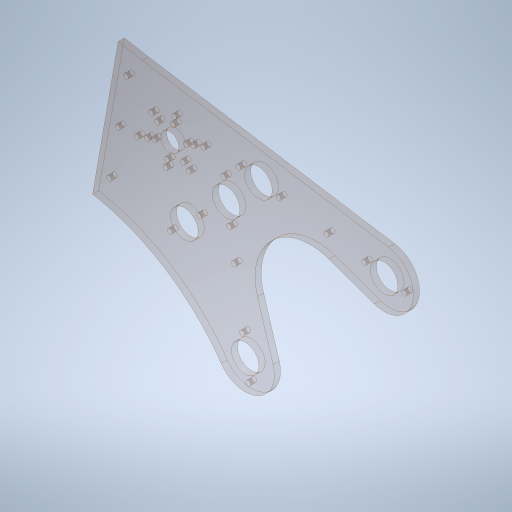
# Autodesk Inventor part: GP7-001
Saved by Autodesk Inventor 2023.4 (Build 274418000, 418)
## iProperties
Created: 2025-02-24
Part Number: GP7-001
Material: Polycarbonate, Smoke
Document SubType Name: Modeling
Designer: dlangdon
Density: 1.2 g/cm^3
Appearance: Polycarbonate - Smoked
Author: dlangdon
Autodesk Inventor part; units mm, degrees
ref_plane "YZ Plane" through (0, 0, 0) normal (1, 0, 0) x (0, 1, 0)
ref_plane "XZ Plane" through (0, 0, 0) normal (0, 1, 0) x (-1, 0, 0)
ref_plane "XY Plane" through (0, 0, 0) normal (0, 0, 1) x (1, 0, 0)
sketch "Sketch1" plane through (0, 0, 0) normal (0, 0, 1) x (1, 0, 0)
  circle A0 centre (71.842, 71.842) radius 50.8 construction
  circle A1 centre (-71.842, -71.842) radius 50.8 construction
  circle A2 centre (0, 0) radius 50.8 construction
  line L0 (-35.921, -35.921) -> (35.921, 35.921) construction
  line L1 (71.842, 71.842) -> (-71.842, -71.842) construction
  line L2 (-4.3707, 6.2419) -> (-4.3707, 50.6116) construction
  line L3 (-226.8798, -122.642) -> (638.5123, -122.642) construction
  circle A3 centre (147.8406, -65.492) radius 57.15 construction
  circle A4 centre (71.842, 71.842) radius 14.2875
  circle A5 centre (-71.842, -71.842) radius 14.2875
  circle A6 centre (-4.3707, 6.2419) radius 57.15 construction
  circle A7 centre (-71.842, -71.842) radius 30.1625 construction
  circle A8 centre (71.842, 71.842) radius 30.1625 construction
  circle A9 centre (-58.1587, 92.2793) radius 14.2875
  line L4 (-58.1587, 92.2793) -> (71.842, 71.842) construction
  circle A10 centre (71.842, 71.842) radius 14.3256 construction
  circle A11 centre (-71.842, -71.842) radius 14.3256 construction
  circle A12 centre (-91.5532, 58.2708) radius 14.2875
  line L5 (-71.842, -71.842) -> (-91.5532, 58.2708) construction
  circle A13 centre (-91.5532, 58.2708) radius 23.8316 construction
  circle A14 centre (-58.1587, 92.2793) radius 23.8316 construction
  line L6 (14.744, 60.1006) -> (61.7538, 43.4167)
  line L7 (-42.9911, -63.0445) -> (-59.0357, -10.4271)
  arc A15 (14.744, 60.1006) -> (-59.0357, -10.4271) centre (-4.3707, 6.2419) ccw
  line L8 (-203.1376, 146.1202) -> (-178.1235, 141.7096)
  line L9 (-178.1235, 141.7096) -> (-204.5875, -8.3751) construction
  line L10 (-204.5875, -8.3751) -> (-229.6016, -3.9645) construction
  line L11 (-229.6016, -3.9645) -> (-203.1376, 146.1202) construction
  line L12 (-245.2736, -92.8451) -> (35.0702, -142.2772) construction
  line L13 (-198.7269, 171.1343) -> (174.1389, 105.388) construction
  line L14 (-198.7269, 171.1343) -> (-245.2736, -92.8451) construction
  circle A16 centre (-149.8604, 82.5886) radius 31.75 construction
  line L15 (-87.9836, 34.7081) -> (-79.4511, -21.6151) construction
  circle A17 centre (12.249, 81.2106) radius 9.525 construction
  line L16 (-190.6305, 143.9149) -> (-217.0945, -6.1698) construction
  line L17 (-195.0412, 118.9008) -> (-212.6839, 18.8443) construction
  circle A18 centre (-149.8604, 82.5886) radius 17.4625 construction
  circle A19 centre (-149.8604, 82.5886) radius 9.525
  circle A20 centre (-58.1587, 92.2793) radius 30.1816 construction
  line L18 (-203.1376, 146.1202) -> (-229.6016, -3.9645)
  arc A21 (61.7538, 43.4167) -> (76.5306, 101.6379) centre (71.842, 71.842) ccw
  arc A22 (-96.6164, -89.047) -> (-42.9911, -63.0445) centre (-71.842, -71.842) ccw
  line L19 (-149.8604, 82.5886) -> (-133.451, 88.5611) construction
  line L20 (-115.5498, 95.0766) -> (-184.1709, 70.1006) construction
  circle A23 centre (-184.1709, 70.1006) radius 4.7625 construction
  line L21 (0, 0) -> (-4.3707, 6.2419) construction
  circle A24 centre (71.842, 71.842) radius 28.6512 construction
  line L22 (64.3298, 44.1932) -> (-61.9049, 78.4917) construction
  line L23 (73.1757, 100.4622) -> (-57.4936, 106.5513) construction
  line L24 (-178.1235, 141.7096) -> (76.5306, 101.6379)
  line L25 (-149.8604, 82.5886) -> (-134.7687, 17.0965) construction
  circle A25 centre (-134.7687, 17.0965) radius 31.75 construction
  circle A26 centre (-134.7687, 17.0965) radius 14.2875
  line L26 (-91.5532, 58.2708) -> (-134.7687, 17.0965) construction
  circle A27 centre (-149.8604, 82.5886) radius 25.4 construction
  arc A28 (-96.6164, -89.047) -> (-229.6016, -3.9645) centre (-265.2541, -206.1602) ccw
  point P0 (-83.7173, 6.5465)
  point P1 (-203.8625, 68.8725)
  point P2 (-203.8625, 68.8725)
  point P3 (-146.828, 99.7858)
  point P4 (-163.2374, 93.8133)
  point P5 (-166.2697, 76.6161)
  point P6 (-152.8927, 65.3914)
  point P7 (-136.4833, 71.3639)
  point P8 (-125.9922, 91.2759)
  point P9 (-145.4497, 107.6027)
  point P10 (-169.3179, 98.9154)
  point P11 (-173.7285, 73.9013)
  point P12 (-154.271, 57.5745)
  point P13 (-130.4028, 66.2618)
  dimension "d7" = 101.6
  dimension "d18" = 47.6631
  dimension "d34" = 34.925
  dimension "d65" = 50.8
  dimension "d3" = 45
  dimension "d4" = 0
  dimension "d8" = 101.6
  dimension "d9" = 28.575
  dimension "d10" = 101.6
  dimension "d11" = 114.3
  dimension "d12" = 114.3
  dimension "d13" = 15.875
  dimension "d14" = 15.875
  dimension "d15" = 131.5974
  dimension "d16" = 28.6512
  dimension "d17" = 131.5974
  dimension "d19" = 47.6631
  dimension "d22" = 25.4
  dimension "d23" = 152.4
  dimension "d26" = 268.0517
  dimension "d27" = 63.5
  dimension "d30" = 200.025
  dimension "d31" = 10
  dimension "d32" = 19.05
  dimension "d33" = 101.6
  dimension "d35" = 19.05
  dimension "d36" = 6.35
  dimension "d40" = 360
  dimension "d44" = 9.525
  dimension "d55" = 80
  dimension "d56" = 7.62
  dimension "d57" = 25.4
  dimension "d58" = 57.3024
  dimension "d59" = 63.5
  dimension "d60" = 67.2084
  dimension "d61" = 59.69
  dimension "d62" = 55
  dimension "d68" = 360
  dimension "d70" = 38.1
  dimension "d71" = 60
  constraints: 54 end point, 25 centre point, 23 coincident, 21 point on circle, 16 tangent, 7 midpoint, 6 equal radius, 5 point on line, 4 collinear, 4 parallel, 2 horizontal, 1 concentric, 1 perpendicular, 1 vertical, 29 other
  measures "d3" angle of L2 L0
  measures "d4" distance between parallel lines of L0 L1
  measures "d8" diameter of A2
  measures "d9" diameter of A4
  measures "d10" diameter of A0
  measures "d11" diameter of A3
  measures "d12" diameter of A6
  measures "d13" radial gap between concentric circles of A5 A7
  measures "d14" radial gap between concentric circles of A4 A8
  measures "d15" distance of L4.start L4.end
  measures "d16" diameter of A10
  measures "d17" distance of L5.start L5.end
  measures "d19" diameter of A14
  measures "d22" distance of L9.end L10.end
  measures "d23" distance of L10.end L8.start
  measures "d26" distance of L13.start L12.start
  measures "d27" diameter of A16
  measures "d30" distance from line of point (0, 0) L9
  measures "d31" angle of L3 L12
  measures "d32" diameter of A17
  measures "d33" distance of L17.start L17.end
  measures "d35" diameter of A19
  measures "d36" radial gap between concentric circles of A14 A20
  measures "d44" diameter of A23
  measures "d55" angle of L1 L21
  measures "d56" distance of L21.start L21.end
  measures "d57" distance between parallel lines of L13 L8
  measures "d58" diameter of A24
  measures "d59" diameter of A25
  measures "d60" distance of L19.start L25.end
  measures "d61" distance of L26.start L26.end
  measures "d62" angle of L15 L26
  measures "d70" distance from line of L9 L19.start
  measures "d71" angle of L9 L20
extrude "Extrusion1" add sketch "Sketch1" along normal blind 6.35
hole "Hole1" at (12.249, 81.2106, 0) at (-195.0412, 118.9008, 0) at (-203.8625, 68.8725, 0) at (-212.6839, 18.8443, 0) at (-133.451, 88.5611, 0) at (-146.828, 99.7858, 0) at (-163.2374, 93.8133, 0) at (-166.2697, 76.6161, 0) at (-152.8927, 65.3914, 0) at (-136.4833, 71.3639, 0) at (-115.5498, 95.0766, 0) at (-184.1709, 70.1006, 0) at (-154.271, 57.5745, 0) at (-173.7285, 73.9013, 0) at (-169.3179, 98.9154, 0) at (-145.4497, 107.6027, 0) at (-125.9922, 91.2759, 0) at (-130.4028, 66.2618, 0) at (-83.7173, 6.5465, 0) direction (0, 0, 1) diameter 5.1054 end through all clearance for "Flat Head Machine Screw (82)" size "#10" standard "Ansi Unified Screw Threads"
sketch "Sketch2" plane through (0, 0, 6.35) normal (0, 0, 1) x (1, 0, 0)
  circle A0 centre (-130.4028, 66.2618) radius 2.5527 construction
  circle A1 centre (-145.4497, 107.6027) radius 2.5527 construction
  circle A2 centre (-173.7285, 73.9013) radius 2.5527 construction
  circle A3 centre (-184.1709, 70.1006) radius 2.5527 construction
  circle A4 centre (-136.4833, 71.3639) radius 2.5527 construction
  circle A5 centre (-166.2697, 76.6161) radius 2.5527 construction
  circle A6 centre (-146.828, 99.7858) radius 2.5527 construction
  circle A7 centre (-212.6839, 18.8443) radius 2.5527 construction
  circle A8 centre (-195.0412, 118.9008) radius 2.5527 construction
  circle A9 centre (12.249, 81.2106) radius 2.5527 construction
  circle A10 centre (-203.8625, 68.8725) radius 2.5527 construction
  circle A11 centre (-133.451, 88.5611) radius 2.5527 construction
  circle A12 centre (-163.2374, 93.8133) radius 2.5527 construction
  circle A13 centre (-152.8927, 65.3914) radius 2.5527 construction
  circle A14 centre (-115.5498, 95.0766) radius 2.5527 construction
  circle A15 centre (-154.271, 57.5745) radius 2.5527 construction
  circle A16 centre (-169.3179, 98.9154) radius 2.5527 construction
  circle A17 centre (-125.9922, 91.2759) radius 2.5527 construction
  circle A18 centre (-83.7173, 6.5465) radius 2.5527 construction
  line L0 (-42.9911, -63.0445) -> (-59.0357, -10.4271) construction
  arc A19 (14.744, 60.1006) -> (-59.0357, -10.4271) centre (-4.3707, 6.2419) ccw construction
  line L1 (14.744, 60.1006) -> (61.7538, 43.4167) construction
  arc A20 (61.7538, 43.4167) -> (76.5306, 101.6379) centre (71.842, 71.842) ccw construction
  line L2 (76.5306, 101.6379) -> (-178.1235, 141.7096) construction
  line L3 (-178.1235, 141.7096) -> (-203.1376, 146.1202) construction
  line L4 (-203.1376, 146.1202) -> (-229.6016, -3.9645) construction
  arc A21 (-96.6164, -89.047) -> (-229.6016, -3.9645) centre (-265.2541, -206.1602) ccw construction
  arc A22 (-96.6164, -89.047) -> (-42.9911, -63.0445) centre (-71.842, -71.842) ccw construction
  circle A23 centre (-91.5532, 58.2708) radius 14.2875 construction
  circle A24 centre (-149.8604, 82.5886) radius 9.525 construction
  circle A25 centre (-134.7687, 17.0965) radius 14.2875 construction
  circle A26 centre (-58.1587, 92.2793) radius 14.2875 construction
  circle A27 centre (-71.842, -71.842) radius 14.2875 construction
  circle A28 centre (71.842, 71.842) radius 14.2875 construction
  line L5 (-74.9903, -51.0607) -> (-68.6938, -92.6234) construction
  line L6 (-149.986, 2.5979) -> (-119.5513, 31.5951) construction
  line L7 (-94.7014, 79.0522) -> (-88.4049, 37.4894) construction
  line L8 (-78.9222, 95.5435) -> (-37.3952, 89.0151) construction
  line L9 (51.0786, 75.1063) -> (92.6055, 68.5778) construction
  circle A29 centre (-91.5532, 58.2708) radius 14.2875 construction
  line L10 (-58.1587, 92.2793) -> (-91.5532, 58.2708) construction
  line L11 (-58.1587, 92.2793) -> (71.842, 71.842) construction
  line L12 (-91.5532, 58.2708) -> (-134.7687, 17.0965) construction
  line L13 (-91.5532, 58.2708) -> (-71.842, -71.842) construction
  point P0 (0, 0)
  dimension "d72" = 42.037
  constraints: 19 end point, 14 coincident, 5 collinear, 5 midpoint, 4 equal length
  measures "d72" distance of L5.start L5.end
hole "Hole2" at (-74.9903, -51.0607, 6.35) at (-119.5513, 31.5951, 6.35) at (-68.6938, -92.6234, 6.35) at (-149.986, 2.5979, 6.35) at (-88.4049, 37.4894, 6.35) at (-94.7014, 79.0522, 6.35) at (-37.3952, 89.0151, 6.35) at (-78.9222, 95.5435, 6.35) at (92.6055, 68.5778, 6.35) at (51.0786, 75.1063, 6.35) direction (0, 0, -1) diameter 5.1054 end through all clearance for "Flat Head Machine Screw (82)" size "#10" standard "Ansi Unified Screw Threads"
body "Solid1"
